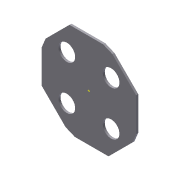
# Autodesk Inventor part: Stage2
Saved by Autodesk Inventor 2018.2 (Build 222227000, 227)
## iProperties
Created: 2018-10-31
Part Number: Stage2
Material: 3.3547 AlMg4,5Mn (AW-5083/H111)
Document SubType Name: Modeling
Designer: N.Grubert
Density: 2.66 g/cm^3
Appearance: Aluminum (gleichmäßig)
Fläche: 0 cm²
Gewicht: 0 g
Material: geeigneten Werkstoff auswählen !
Dateiname: P:\INVENTOR\Inventor 2018\Templates\ILT\Norm.ipt
Bez_eng: bolt
Bez_french: boulon
Author: N.Grubert
Autodesk Inventor part; units mm, degrees
ref_plane "YZ Plane" through (0, 0, 0) normal (1, 0, 0) x (0, 1, 0)
ref_plane "XZ Plane" through (0, 0, 0) normal (0, 1, 0) x (-1, 0, 0)
ref_plane "XY Plane" through (0, 0, 0) normal (0, 0, 1) x (1, 0, 0)
sketch "Skizze4" plane through (0, 0, 0) normal (0, 1, 0) x (-1, 0, 0)
  line L0 (-23.4031, 56.5) -> (23.4031, 56.5)
  line L1 (23.4031, 56.5) -> (56.5, 23.4031)
  line L2 (56.5, 23.4031) -> (56.5, -23.4031)
  line L3 (56.5, -23.4031) -> (23.4031, -56.5)
  line L4 (23.4031, -56.5) -> (-23.4031, -56.5)
  line L5 (-23.4031, -56.5) -> (-56.5, -23.4031)
  line L6 (-56.5, -23.4031) -> (-56.5, 23.4031)
  line L7 (-56.5, 23.4031) -> (-23.4031, 56.5)
  line L8 (79.1, 0) -> (-79.1, 0) construction
  line L9 (0, -79.1) -> (0, 79.1) construction
  circle A0 centre (-26.5, 26.5) radius 10
  circle A1 centre (-26.5, -26.5) radius 10
  circle A2 centre (26.5, -26.5) radius 10
  circle A3 centre (26.5, 26.5) radius 10
  point P0 (0, 0)
  point P1 (0, 0)
  dimension "d4" = 113
  dimension "d5" = 20
  dimension "d6" = 30
  dimension "d7" = 30
  dimension "d10" = 360
  constraints: 16 end point, 4 centre point, 1 coincident, 28 other
  measures "d4" distance between parallel lines of L4 L0
  measures "d5" diameter of A0
  measures "d6" distance from line of A0.centre L6
  measures "d7" distance from line of A0.centre L0
extrude "Extrusion2" add sketch "Skizze4" along normal blind 2.5
sketch "Skizze5" plane through (0, 0, 0) normal (0, -1, 0) x (1, 0, 0)
  circle A0 centre (-26.5, 26.5) radius 10 construction
  circle A1 centre (-26.5, -26.5) radius 10 construction
  circle A2 centre (26.5, -26.5) radius 10 construction
  circle A3 centre (26.5, 26.5) radius 10 construction
  line L0 (23.4031, 56.5) -> (-23.4031, 56.5) construction
  line L1 (-23.4031, 56.5) -> (-56.5, 23.4031) construction
  line L2 (-56.5, 23.4031) -> (-56.5, -23.4031) construction
  line L3 (-56.5, -23.4031) -> (-23.4031, -56.5) construction
  line L4 (-23.4031, -56.5) -> (23.4031, -56.5) construction
  line L5 (23.4031, -56.5) -> (56.5, -23.4031) construction
  line L6 (56.5, -23.4031) -> (56.5, 23.4031) construction
  line L7 (56.5, 23.4031) -> (23.4031, 56.5) construction
  line L8 (23.4031, 56.5) -> (56.5, 23.4031) construction
  line L9 (-56.5, -23.4031) -> (-56.5, 23.4031) construction
  line L10 (-23.4031, -56.5) -> (-56.5, -23.4031) construction
  line L11 (23.4031, -56.5) -> (-23.4031, -56.5) construction
  line L12 (56.5, 23.4031) -> (56.5, -23.4031) construction
  line L13 (-56.5, 16.9087) -> (-51.9078, 27.9953)
  line L14 (-56.5, 23.4031) -> (-23.4031, 56.5) projected
  line L15 (-56.5, 23.4031) -> (-56.5, -23.4031) projected
  line L16 (-56.5, 23.4031) -> (-51.9078, 27.9953)
  line L17 (-23.4031, 56.5) -> (-56.5, 23.4031) projected
  line L18 (-56.5, 23.4031) -> (-56.5, 16.9087)
  line L19 (-23.4031, -56.5) -> (-27.9953, -51.9078)
  line L20 (-16.9087, -56.5) -> (-27.9953, -51.9078)
  line L21 (-23.4031, -56.5) -> (-16.9087, -56.5)
  line L22 (56.5, -23.4031) -> (51.9078, -27.9953)
  line L23 (56.5, -16.9087) -> (51.9078, -27.9953)
  line L24 (56.5, -23.4031) -> (56.5, -16.9087)
  line L25 (23.4031, 56.5) -> (27.9953, 51.9078)
  line L26 (16.9087, 56.5) -> (27.9953, 51.9078)
  line L27 (23.4031, 56.5) -> (16.9087, 56.5)
  point P0 (0, 0)
  dimension "d21" = 22.5
  dimension "d22" = 12
  dimension "d25" = 360
  constraints: 24 end point, 4 coincident, 2 collinear, 2 point on line, 25 other
  measures "d21" angle of L13 L1
  measures "d22" distance of L13.start L13.end
extrude "Extrusion3" cut sketch "Skizze5" against normal blind 10
equation "\"d7\" = d6"
